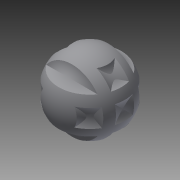
# Autodesk Inventor part: Ball Concept1
Saved by Autodesk Inventor 2015 (Build 190159000, 159)
## iProperties
Created: 2016-04-09
Part Number: Ball Concept1
Material: Generic
Document SubType Name: Modeling
Designer: tquinn
Density: 1 g/cm^3
Appearance: Default
Author: tquinn
Autodesk Inventor part; units mm, degrees
ref_plane "YZ Plane" through (0, 0, 0) normal (1, 0, 0) x (0, 1, 0)
ref_plane "XZ Plane" through (0, 0, 0) normal (0, 1, 0) x (-1, 0, 0)
ref_plane "XY Plane" through (0, 0, 0) normal (0, 0, 1) x (1, 0, 0)
sketch "Sketch1" plane through (0, 0, 0) normal (0, 0, 1) x (1, 0, 0)
  circle A0 centre (0, 0) radius 6.35
  line L0 (0, 6.35) -> (0, -6.35)
  line L1 (-6.35, 0) -> (6.35, 0)
  line L2 (0, 6.35) -> (6.35, 6.35)
  line L3 (0, -6.35) -> (6.35, -6.35)
  line L4 (6.35, -6.35) -> (6.35, 0)
  line L5 (0, -6.35) -> (-6.35, -6.35)
  line L6 (-6.35, -6.35) -> (-6.35, 0)
  line L7 (-6.35, 0) -> (-6.35, 6.35)
  line L8 (0, 6.35) -> (-6.35, 6.35)
  line L9 (6.35, 6.35) -> (6.35, 0)
  line L10 (6.35, 3.175) -> (-6.35, 3.175)
  line L11 (6.35, -3.175) -> (-6.35, -3.175)
  line L12 (-3.175, 6.35) -> (-3.175, -6.35)
  line L13 (3.175, -6.35) -> (3.175, 6.35)
  arc A1 (3.175, 5.4993) -> (5.4993, 3.175) centre (6.35, 6.35) ccw
  arc A2 (-5.4993, 3.175) -> (-3.175, 5.4993) centre (-6.3415, 6.3415) ccw
  arc A3 (-3.175, -5.4993) -> (-5.4993, -3.175) centre (-6.3415, -6.3415) ccw
  arc A4 (5.4993, -3.175) -> (3.175, -5.4993) centre (6.3415, -6.3415) ccw
  line L14 (6.35, 3.175) -> (6.35, 0)
  line L15 (6.35, 1.5875) -> (3.175, 1.5875)
  line L16 (6.35, 0) -> (6.35, -3.175)
  line L17 (6.35, -1.5875) -> (3.175, -1.5875)
  arc A5 (6.1484, 1.5875) -> (6.1484, -1.5875) centre (9.0147, 0) ccw
  line L18 (3.175, 1.5875) -> (-6.1484, 1.5875)
  line L19 (3.175, -1.5875) -> (-6.1484, -1.5875)
  arc A6 (-6.1484, -1.5875) -> (-6.1484, 1.5875) centre (-9.0147, 0) ccw
  dimension "d1" = 12.7
  dimension "d13" = 3.2766
  dimension "d14" = 3.2766
  dimension "d15" = 3.2766
  dimension "d16" = 3.2766
  dimension "d17" = 3.2766
  constraints: 40 end point, 15 point on line, 12 point on circle, 10 midpoint, 7 horizontal, 7 vertical, 6 centre point, 5 perpendicular, 2 coincident, 2 collinear, 1 parallel, 18 other
  measures "d13" radius of A2
  measures "d14" radius of A3
  measures "d15" radius of A4
  measures "d16" radius of A5
  measures "d17" radius of A6
revolve "Revolution1" add sketch "Sketch1" angle 360 about axis through (0, 6.35, 0) along (0, -1, 0) contours L15 L13 L10 A0 | A5 L1 L13 L15 | A0 L11 L13 L17 | L17 L13 L1 A5 | L10 L13 A1 | L18 L0 L10 L13 | L13 L1 L0 L18 | A4 L13 L11 | L19 L0 L1 L13 | L13 L11 L0 L19 | L13 L10 L0 A0 | A0 L0 L11 L13
sketch "Sketch3" plane through (0, 0, 0) normal (0, 1, 0) x (-1, 0, 0)
  circle A0 centre (0, 0) radius 6.35
  line L0 (0, 6.35) -> (0, -6.35)
  line L1 (-6.35, 0) -> (6.35, 0)
  line L2 (0, 6.35) -> (6.35, 6.35)
  line L3 (0, -6.35) -> (6.35, -6.35)
  line L4 (6.35, -6.35) -> (6.35, 0)
  line L5 (0, -6.35) -> (-6.35, -6.35)
  line L6 (-6.35, -6.35) -> (-6.35, 0)
  line L7 (-6.35, 0) -> (-6.35, 6.35)
  line L8 (0, 6.35) -> (-6.35, 6.35)
  line L9 (6.35, 6.35) -> (6.35, 0)
  line L10 (6.35, 3.175) -> (-6.35, 3.175)
  line L11 (6.35, -3.175) -> (-6.35, -3.175)
  line L12 (-3.175, 6.35) -> (-3.175, -6.35)
  line L13 (3.175, -6.35) -> (3.175, 6.35)
  arc A1 (3.175, 5.4993) -> (5.4993, 3.175) centre (6.35, 6.35) ccw
  arc A2 (-5.4993, 3.175) -> (-3.175, 5.4993) centre (-6.3415, 6.3415) ccw
  arc A3 (-3.175, -5.4993) -> (-5.4993, -3.175) centre (-6.3415, -6.3415) ccw
  arc A4 (5.4993, -3.175) -> (3.175, -5.4993) centre (6.3415, -6.3415) ccw
  line L14 (6.35, 3.175) -> (6.35, 0)
  line L15 (6.35, 1.5875) -> (3.175, 1.5875)
  line L16 (6.35, 0) -> (6.35, -3.175)
  line L17 (6.35, -1.5875) -> (3.175, -1.5875)
  arc A5 (6.1484, 1.5875) -> (6.1484, -1.5875) centre (9.0147, 0) ccw
  line L18 (3.175, 1.5875) -> (-6.1484, 1.5875)
  line L19 (3.175, -1.5875) -> (-6.1484, -1.5875)
  arc A6 (-6.1484, -1.5875) -> (-6.1484, 1.5875) centre (-9.0147, 0) ccw
  dimension "d18" = 12.7
  dimension "d19" = 3.2766
  dimension "d20" = 3.2766
  dimension "d21" = 3.2766
  dimension "d22" = 3.2766
  dimension "d23" = 3.2766
  constraints: 40 end point, 15 point on line, 12 point on circle, 10 midpoint, 7 horizontal, 7 vertical, 6 centre point, 5 perpendicular, 2 coincident, 2 collinear, 1 parallel, 18 other
  measures "d19" radius of A2
  measures "d20" radius of A3
  measures "d21" radius of A4
  measures "d22" radius of A5
  measures "d23" radius of A6
revolve "Revolution2" add sketch "Sketch3" angle 360 about axis through (0, 0, 6.35) along (0, 0, -1) contours L18 L12 L10 L0 | L0 L1 L12 L18 | L19 L12 L1 L0 | L0 L11 L12 L19 | L0 L10 L12 A0 | L18 A0 L10 L12 | L12 L1 A6 L18 | A0 L12 L11 L0 | L19 A6 L1 L12 | L12 L11 A0 L19 | L12 L10 A2 | A3 L11 L12
body "Solid1"
